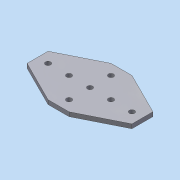
# Autodesk Inventor part: 7 Hole Cross Joining Plate
Saved by Autodesk Inventor 2013 (Build 170138000, 138)
## iProperties
Created: 2013-12-08
Part Number: 7 Hole Cross Joining Plate
Material: Aluminum 6061
Document SubType Name: Modeling
Density: 2.71 g/cm^3
Catalog Web Link: www.openbuildspartstore.com
Vendor: OpenBuilds
Mass: 46.2061 g
Surface Area: 100.005 cm^2
Volume: 17.0502 cm^3
Author: Work
Autodesk Inventor part; units mm, degrees
ref_plane "YZ Plane" through (0, 0, 0) normal (1, 0, 0) x (0, 1, 0)
ref_plane "XZ Plane" through (0, 0, 0) normal (0, 1, 0) x (-1, 0, 0)
ref_plane "XY Plane" through (0, 0, 0) normal (0, 0, 1) x (1, 0, 0)
sketch "Sketch1" plane through (0, 0, 0) normal (0, 0, 1) x (1, 0, 0)
  line L0 (-50, 10) -> (50, 10) construction
  line L1 (50, 10) -> (50, -10) construction
  line L2 (50, -10) -> (-50, -10) construction
  line L3 (-50, -10) -> (-50, 10) construction
  line L4 (-50, 10) -> (50, -10) construction
  line L5 (50, 10) -> (-50, -10) construction
  line L6 (10, -30) -> (-10, -30) construction
  line L7 (-10, -30) -> (-10, 30) construction
  line L8 (-10, 30) -> (10, 30) construction
  line L9 (10, 30) -> (10, -30) construction
  line L10 (10, -30) -> (-10, 30) construction
  line L11 (-10, -30) -> (10, 30) construction
  line L12 (-50, 10) -> (-10, 30)
  line L13 (-10, 30) -> (10, 30)
  line L14 (10, 30) -> (50, 10)
  line L15 (50, 10) -> (50, -10)
  line L16 (50, -10) -> (10, -30)
  line L17 (10, -30) -> (-10, -30)
  line L18 (-10, -30) -> (-50, -10)
  line L19 (-50, -10) -> (-50, 10)
  point P0 (0, 0)
  dimension "d0" = 20
  dimension "d2" = 100
  dimension "d3" = 20
  dimension "d4" = 60
  constraints: 40 end point, 10 equal length, 4 midpoint, 2 horizontal, 2 perpendicular
  measures "d0" distance of L0.end L1.end
  measures "d2" distance of L1.end L2.end
  measures "d3" distance of L6.start L6.end
  measures "d4" distance of L8.end L6.start
extrude "Extrusion1" add sketch "Sketch1" along normal mid plane 4
sketch "Sketch2" plane through (0, 0, 2) normal (0, 0, 1) x (1, 0, 0)
  line L0 (-50, 10) -> (-50, -10) projected
  line L1 (-10, -30) -> (10, -30) projected
  line L2 (50, -10) -> (50, 10) projected
  line L3 (10, 30) -> (-10, 30) projected
  line L4 (0, 30) -> (0, -30) construction
  line L5 (-50, 0) -> (50, 0) construction
  point P0 (0, 0)
  point P1 (0, 0)
  point P2 (20, 0)
  point P3 (40, 0)
  point P4 (0, 20)
  point P5 (0, -20)
  point P6 (-20, 0)
  point P7 (-40, 0)
  dimension "d7" = 20
  dimension "d9" = 20
  dimension "d10" = 20
  dimension "d11" = 20
  dimension "d12" = 20
  dimension "d13" = 20
  constraints: 6 point on line, 4 end point, 4 midpoint, 1 coincident
  measures "d7" distance of point (20, 0) point (0, 0)
  measures "d9" distance of point (40, 0) point (20, 0)
  measures "d10" distance of point (0, 0) point (0, -20)
  measures "d11" distance of point (-20, 0) point (0, 0)
  measures "d12" distance of point (-40, 0) point (-20, 0)
  measures "d13" distance of point (0, 20) point (0, 0)
hole "Hole1" at (0, 0, 2) at (20, 0, 2) at (40, 0, 2) at (0, 20, 2) at (0, -20, 2) at (-20, 0, 2) at (-40, 0, 2) direction (0, 0, -1) diameter 5 end through all
equation "\"d9\" = d7"
equation "\"d10\" = d7"
equation "\"d11\" = d10"
equation "\"d12\" = d11"
equation "\"d13\" = d10"
body "Solid1"
